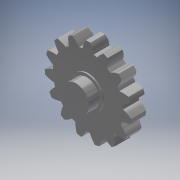
# Autodesk Inventor part: Spur Gear1
Saved by Autodesk Inventor 2019.4 (Build 234330000, 330)
## iProperties
Created: 2020-02-16
Part Number: Spur Gear1
Material: Steel
Document SubType Name: Modeling
Designer: admin
Categories: <?xml version="1.0" encoding="UTF-16"?> <MemberInstance><Categories><FamilyTemplate><FamilyTemplateParameter ValueType="xs:double" Id="1" ObjectReferenceKey="da_z" ObjectType="kUserParameterObject"/><FamilyTemplateParameter ValueType="xs:double" Id="2" ObjectReferenceKey="da_b" ObjectType="kUserParameterObject"/><FamilyTemplateParameter ValueType="xs:double" Id="3" ObjectReferenceKey="da_beta" ObjectType="kUserParameterObject"/><FamilyTemplateParameter ValueType="xs:double" Id="4" ObjectReferenceKey="da_da" ObjectType="kUserParameterObject"/><FamilyTemplateParameter ValueType="xs:double" Id="5" ObjectReferenceKey="da_aw" ObjectType="kUserParameterObject"/><FamilyTemplateParameter ValueType="xs:string" Id="6" ObjectReferenceKey="EAIAABAAAACIAQAAAAAAAIAAAAAAAAAA" ObjectType="83910656" SubObjectId="SurfaceGeometry"/></FamilyTemplate><ParamToTemplateMap><ParamToTemplate CategoryParameter="//CategoryParameter[@InternalName='046C89C9-8512-4d59-83FE-43B91F4F132A']" TemplateParameter="1"/><ParamToTemplate CategoryParameter="//CategoryParameter[@InternalName='2552DF32-E462-4b46-AEBF-C6C7768E72AC']" TemplateParameter="2"/><ParamToTemplate CategoryParameter="//CategoryParameter[@InternalName='C9EE641D-15FC-4fae-A226-E94C4372FDD7']" TemplateParameter="3"/><ParamToTemplate><ParamToTemplate CategoryParameter="//CategoryParameter[@InternalName='00B6519A-459B-49c7-AD84-2E56D39A5744']" ConstantValue="0.300000"/></ParamToTemplate><ParamToTemplate><ParamToTemplate CategoryParameter="//CategoryParameter[@InternalName='04B31F0E-C7A6-4894-AA32-9629BEFACF47']" ConstantValue="0.400000"/></ParamToTemplate><ParamToTemplate><ParamToTemplate CategoryParameter="//CategoryParameter[@InternalName='43CBEC2E-7847-49e7-A936-2F7889FCB2D9']" ConstantValue="0.800000"/></ParamToTemplate><ParamToTemplate><ParamToTemplate CategoryParameter="//CategoryParameter[@InternalName='B1EFC894-105D-4ebd-86BF-FA20ED196853']" ConstantValue="0.900000"/></ParamToTemplate><ParamToTemplate><ParamToTemplate CategoryParameter="//CategoryParameter[@InternalName='51175063-3D10-4879-93E8-6246FE8B403D']" ConstantValue="2060000000.000000"/></ParamToTemplate><ParamToTemplate><ParamToTemplate CategoryParameter="//CategoryParameter[@InternalName='A3A52E27-4454-46a9-B0BD-C932399B70AF']" ConstantValue="0.300000"/></ParamToTemplate><ParamToTemplate><ParamToTemplate CategoryParameter="//CategoryParameter[@InternalName='91B76062-C214-41d9-B1B9-14D2AB99603D']" ConstantValue="0.200000"/></ParamToTemplate><ParamToTemplate><ParamToTemplate CategoryParameter="//CategoryParameter[@InternalName='374E806E-8B8A-4dda-A9AA-1039D6500AD2']" ConstantValue="5.000000"/></ParamToTemplate><ParamToTemplate><ParamToTemplate CategoryParameter="//CategoryParameter[@InternalName='2D373A89-B862-43d6-8D0B-0CBF12AB9F6C']" ConstantValue="0.349066"/></ParamToTemplate><ParamToTemplate CategoryParameter="//CategoryParameter[@InternalName='37777632-D6A2-4fac-9D53-DB8ACD95C989']" TemplateParameter="4"/><ParamToTemplate CategoryParameter="//CategoryParameter[@InternalName='FD1017F1-B727-4f7e-9707-0F86F1FF9423']" TemplateParameter="5"/><ParamToTemplate><ParamToTemplate CategoryParameter="//CategoryParameter[@InternalName='9E1B4470-B2D3-4ff1-B813-535BB4CDF51A']" ConstantValue="3520000.000000"/></ParamToTemplate><ParamToTemplate><ParamToTemplate CategoryParameter="//CategoryParameter[@InternalName='F8452263-BFF6-458c-9FB1-07C4B99E95CD']" ConstantValue="11400000.000000"/></ParamToTemplate><ParamToTemplate><ParamToTemplate CategoryParameter="//CategoryParameter[@InternalName='3E3BB259-FD49-497f-8171-6EBC954A3479']" ConstantValue="2.000000"/></ParamToTemplate><ParamToTemplate CategoryParameter="//CategoryParameter[@InternalName='27C3BAF2-7550-4e4b-AE2C-0DB134B7D9B7']" TemplateParameter="6"/></ParamToTemplateMap><Category DisplayName="Gear" InternalName="DC85795E-93AB-48d5-8EEE-5A27447B64BD" Mnemonic="Gear"><CategoryParameter DisplayName="z" InternalName="046C89C9-8512-4d59-83FE-43B91F4F132A" Mnemonic="z"/><CategoryParameter DisplayName="b" InternalName="2552DF32-E462-4b46-AEBF-C6C7768E72AC" Mnemonic="b"/><CategoryParameter DisplayName="||b|" InternalName="C9EE641D-15FC-4fae-A226-E94C4372FDD7" Mnemonic="beta"/><CategoryParameter DisplayName="x" InternalName="00B6519A-459B-49c7-AD84-2E56D39A5744" Mnemonic="x"/><CategoryParameter DisplayName="a*" InternalName="04B31F0E-C7A6-4894-AA32-9629BEFACF47" Mnemonic="a"/><CategoryParameter DisplayName="c*" InternalName="43CBEC2E-7847-49e7-A936-2F7889FCB2D9" Mnemonic="c"/><CategoryParameter DisplayName="r|.f|*" InternalName="B1EFC894-105D-4ebd-86BF-FA20ED196853" Mnemonic="rf"/><CategoryParameter DisplayName="E" InternalName="51175063-3D10-4879-93E8-6246FE8B403D" Mnemonic="E"/><CategoryParameter DisplayName="||m|" InternalName="A3A52E27-4454-46a9-B0BD-C932399B70AF" Mnemonic="mi"/><Category DisplayName="SpurGear" InternalName="26C5A22E-A91E-4dfd-A3B3-23CCAFAE1764" Mnemonic="SpurGear"><CategoryParameter DisplayName="m" InternalName="91B76062-C214-41d9-B1B9-14D2AB99603D" Mnemonic="m"/><CategoryParameter DisplayName="P" InternalName="374E806E-8B8A-4dda-A9AA-1039D6500AD2" Mnemonic="PP"/><CategoryParameter DisplayName="||a|" InternalName="2D373A89-B862-43d6-8D0B-0CBF12AB9F6C" Mnemonic="alpha"/><CategoryParameter DisplayName="d|.a|" InternalName="37777632-D6A2-4fac-9D53-DB8ACD95C989" Mnemonic="da"/><CategoryParameter DisplayName="a|.w|" InternalName="FD1017F1-B727-4f7e-9707-0F86F1FF9423" Mnemonic="aw"/><CategoryParameter DisplayName="||s||.Flim|" InternalName="9E1B4470-B2D3-4ff1-B813-535BB4CDF51A" Mnemonic="sFlim"/><CategoryParameter DisplayName="||s||.Hlim|" InternalName="F8452263-BFF6-458c-9FB1-07C4B99E95CD" Mnemonic="sHlim"/><CategoryParameter DisplayName="type" InternalName="3E3BB259-FD49-497f-8171-6EBC954A3479" Mnemonic="type"/><CategoryParameter DisplayName="PitchDiameter" InternalName="27C3BAF2-7550-4e4b-AE2C-0DB134B7D9B7" Mnemonic="IDS_PITCHDIAM"/></Category></Category></Categories></MemberInstance>
Density: 1 g/cm^3
Appearance: Steel
CustomPartVersion: 1
Author: admin
Autodesk Inventor part; units mm, degrees
sketch "Sketch1" plane through (0, 0, 0) normal (0, 0, 1) x (1, 0, 0)
  circle A0 centre (0, 0) radius 16.2859
  dimension "d0" = 32.5719
  constraints: 1 centre point
  measures "d0" diameter of A0
extrude "Extrusion1" add sketch "Sketch1" along normal blind 6
ref_plane "Work Plane2" through (0, 0, 3) normal (0, 0, 1) x (1, 0, 0)
sketch "Sketch2" plane through (0, 0, 0) normal (0, 0, -1) x (-1, 0, 0)
  circle A0 centre (0, 0) radius 16.2859 projected
  circle A1 centre (0, 0) radius 15.5016
  dimension "d3" = 31.0031
  constraints: 1 centre point, 1 coincident
  measures "d3" diameter of A1
surface extrude "Pitch Diameter" sketch "Sketch2" against normal through all shown no curves A1
ref_plane "Work Plane8" through (0, 0, 0) normal (0.9781476, 0.2079117, 0) x (0, 0, 1)
ref_plane "Work Plane9" through (0, 0, 0) normal (1, 0, 0) x (0, 1, 0)
spur gear teeth "Spur Gear" teeth 15 pitch diameter 30 tip diameter 32.5719 root diameter 26.4 face width 6 start plane through (0, 0, 0) normal (0, 0, -1) x (-1, 0, 0)
sketch "Sketch3" plane through (0, 0, 0) normal (0, 1, 0) x (-1, 0, 0)
  line L0 (16.4963, 0.5) -> (14.7636, 0)
  line L1 (14.7636, 0) -> (17.15, -0.599)
  line L2 (17.15, -0.599) -> (17.9681, 0.8017)
  line L3 (17.9681, 0.8017) -> (16.4963, 0.5)
  line L4 (7.1892, 0) -> (7.3937, 0) projected
  line L5 (7.3937, 0) -> (5.8364, 0) projected
  line L6 (5.8364, 0) -> (3.4164, 0) projected
  line L7 (3.4164, 0) -> (2.0649, 0) projected
  line L8 (2.0649, 0) -> (0.8523, 0) projected
  line L9 (0.8523, 0) -> (-0.8523, 0) projected
  line L10 (-0.8523, 0) -> (-2.0649, 0) projected
  line L11 (-2.0649, 0) -> (-3.4164, 0) projected
  line L12 (-3.4164, 0) -> (-5.8364, 0) projected
  line L13 (-5.8364, 0) -> (-7.3937, 0) projected
  line L14 (-7.3937, 0) -> (-7.1892, 0) projected
  line L15 (-7.1892, 0) -> (-8.307, 0) projected
  line L16 (-8.307, 0) -> (-11.5159, 0) projected
  line L17 (-11.5159, 0) -> (-12.6565, 0) projected
  line L18 (-12.6565, 0) -> (-11.0705, 0) projected
  line L19 (-11.0705, 0) -> (-11.7613, 0) projected
  line L20 (-11.7613, 0) -> (-15.2042, 0) projected
  line L21 (-15.2042, 0) -> (-15.731, 0) projected
  line L22 (-15.731, 0) -> (-13.0375, 0) projected
  line L23 (-13.0375, 0) -> (-13.1819, 0) projected
  line L24 (-13.1819, 0) -> (-16.2636, 0) projected
  line L25 (-16.2636, 0) -> (-16.0854, 0) projected
  line L26 (-16.0854, 0) -> (-12.7502, 0) projected
  line L27 (-12.7502, 0) -> (-12.3233, 0) projected
  line L28 (-12.3233, 0) -> (-14.5109, 0) projected
  line L29 (-14.5109, 0) -> (-13.6585, 0) projected
  line L30 (-13.6585, 0) -> (-10.2583, 0) projected
  line L31 (-10.2583, 0) -> (-9.3338, 0) projected
  line L32 (-9.3338, 0) -> (-10.2491, 0) projected
  line L33 (-10.2491, 0) -> (-8.87, 0) projected
  line L34 (-8.87, 0) -> (-5.9927, 0) projected
  line L35 (-5.9927, 0) -> (-4.7305, 0) projected
  line L36 (-4.7305, 0) -> (-4.2151, 0) projected
  line L37 (-4.2151, 0) -> (-2.5477, 0) projected
  line L38 (-2.5477, 0) -> (-0.6908, 0) projected
  line L39 (-0.6908, 0) -> (0.6908, 0) projected
  line L40 (0.6908, 0) -> (2.5477, 0) projected
  line L41 (2.5477, 0) -> (4.2151, 0) projected
  line L42 (4.2151, 0) -> (4.7305, 0) projected
  line L43 (4.7305, 0) -> (5.9927, 0) projected
  line L44 (5.9927, 0) -> (8.87, 0) projected
  line L45 (8.87, 0) -> (10.2491, 0) projected
  line L46 (10.2491, 0) -> (9.3338, 0) projected
  line L47 (9.3338, 0) -> (10.2583, 0) projected
  line L48 (10.2583, 0) -> (13.6585, 0) projected
  line L49 (13.6585, 0) -> (14.5109, 0) projected
  line L50 (14.5109, 0) -> (12.3233, 0) projected
  line L51 (12.3233, 0) -> (12.7502, 0) projected
  line L52 (12.7502, 0) -> (16.0854, 0) projected
  line L53 (16.0854, 0) -> (16.2636, 0) projected
  line L54 (16.2636, 0) -> (13.1819, 0) projected
  line L55 (13.1819, 0) -> (13.0375, 0) projected
  line L56 (13.0375, 0) -> (15.731, 0) projected
  line L57 (15.731, 0) -> (11.7613, 0) projected
  line L58 (11.7613, 0) -> (11.0705, 0) projected
  line L59 (11.0705, 0) -> (11.0705, 0) projected
  line L60 (11.0705, 0) -> (12.6565, 0) projected
  line L61 (12.6565, 0) -> (11.5159, 0) projected
  line L62 (11.5159, 0) -> (8.307, 0) projected
  line L63 (8.307, 0) -> (7.1892, 0) projected
  line L64 (11.0705, 0) -> (11.7613, 0) projected
  line L65 (16.2636, 6) -> (16.2636, 0) projected
  line L66 (0, 0) -> (0, 13.0925) construction
  dimension "d49" = 0.5
  dimension "d50" = 1.5
  constraints: 10 end point, 1 vertical, 2 other
  measures "d49" vertical distance of L0.start L0.end
  measures "d50" distance of L53.end L0.end
revolve "Revolution1" cut sketch "Sketch3" angle 360 about axis through (0, 0, 0) along (0, 0, 1)
sketch "Sketch4" plane through (0, 0, 6) normal (0, 0, 1) x (1, 0, 0)
  circle A0 centre (0, 0) radius 6
  dimension "d52" = 12
  constraints: 1 centre point, 1 coincident
  measures "d52" diameter of A0
extrude "Extrusion2" add sketch "Sketch4" along normal blind 0.5
sketch "Sketch5" plane through (0, 0, 6.5) normal (0, 0, 1) x (1, 0, 0)
  circle A0 centre (0, 0) radius 4.9
  dimension "d55" = 9.8
  constraints: 1 centre point, 1 coincident
  measures "d55" diameter of A0
extrude "Extrusion3" add sketch "Sketch5" along normal blind 4
equation "\"d0\" = da_da"
equation "\"d1\" = da_b"
equation "\"d3\" = da_dw"
equation "\"d16\" = da_aw"
equation "\"d43\" = da_aw"
equation "\"d46\" = da_aw"
equation "\"da_da\" = 32.571867"
equation "\"da_b\" = 6"
equation "\"da_dw\" = 31.003145"
equation "\"da_aw\" = 31.003145"
body "Solid1"
body "Srf1"
